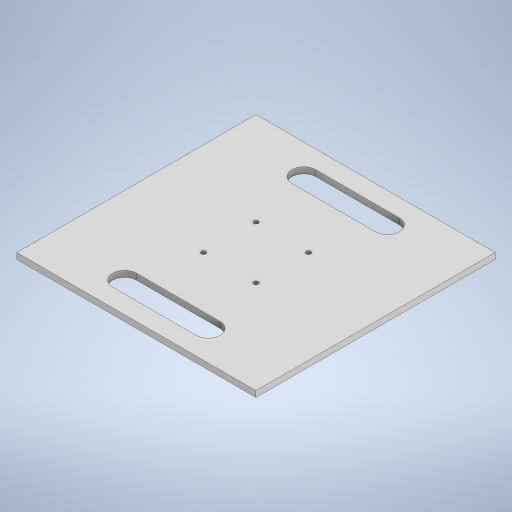
# Autodesk Inventor part: Base myCobot
Saved by Autodesk Inventor 2023.1 (Build 271208000, 208)
## iProperties
Created: 2023-04-03
Part Number: Base myCobot
Material: Generic
Document SubType Name: Modeling
Designer: NITRO 5
Density: 1 g/cm^3
Appearance: Default
Author: NITRO 5
## iProperties of the stored document Base myCobot_3DPrint.ipt
Created: 2023-04-04
Part Number: Base myCobot_3DPrint
Material: Generic
Document SubType Name: Modeling
Designer: NITRO 5
Density: 1 g/cm^3
Appearance: Default
Author: NITRO 5
Autodesk Inventor part; units mm, degrees
ref_plane "YZ Plane" through (0, 0, 0) normal (1, 0, 0) x (0, 1, 0)
ref_plane "XZ Plane" through (0, 0, 0) normal (0, 1, 0) x (-1, 0, 0)
ref_plane "XY Plane" through (0, 0, 0) normal (0, 0, 1) x (1, 0, 0)
sketch "Sketch1" plane through (0, 0, 0) normal (0, 1, 0) x (-1, 0, 0)
  line L0 (-100, 100) -> (100, 100)
  line L1 (100, 100) -> (100, -100)
  line L2 (100, -100) -> (-100, -100)
  line L3 (-100, -100) -> (-100, 100)
  line L4 (-100, 100) -> (100, -100) construction
  line L5 (100, 100) -> (-100, -100) construction
  point P0 (0, 0)
  dimension "d0" = 200
  dimension "d1" = 200
  constraints: 12 end point, 2 midpoint, 2 parallel, 1 horizontal, 1 perpendicular
  measures "d0" distance of L1.end L2.end
  measures "d1" distance of L0.end L1.end
extrude "Extrusion1" add sketch "Sketch1" along normal blind 5
sketch "Sketch6" plane through (0, 0, 0) normal (0, -1, 0) x (1, 0, 0)
  line L0 (-22, 22) -> (22, 22)
  line L1 (22, 22) -> (22, -22)
  line L2 (22, -22) -> (-22, -22)
  line L3 (-22, -22) -> (-22, 22)
  line L4 (-22, 22) -> (22, -22) construction
  line L5 (22, 22) -> (-22, -22) construction
  point P0 (0, 0)
  dimension "d10" = 44
  dimension "d11" = 44
  constraints: 12 end point, 4 coincident, 2 midpoint, 2 parallel, 1 horizontal, 1 perpendicular
  measures "d10" distance of L1.end L2.end
  measures "d11" distance of L0.end L1.end
hole "Hole1" at (22, 0, 22) at (22, 0, -22) at (-22, 0, -22) at (-22, 0, 22) direction (0, 1, 0) diameter 4 depth 49.3
sketch "Sketch7" plane through (0, 0, 0) normal (0, -1, 0) x (1, 0, 0)
  circle A0 centre (-22, 22) radius 2 projected
  circle A1 centre (-22, 22) radius 3
  circle A2 centre (22, 22) radius 2 projected
  circle A3 centre (22, 22) radius 3
  circle A4 centre (-22, -22) radius 2 projected
  circle A5 centre (-22, -22) radius 3
  circle A6 centre (22, -22) radius 3
  point P0 (0, 0)
  dimension "d19" = 6
  dimension "d20" = 6
  dimension "d21" = 6
  dimension "d22" = 6
  constraints: 4 centre point, 3 coincident
  measures "d19" diameter of A1
  measures "d20" diameter of A3
  measures "d21" diameter of A5
  measures "d22" diameter of A6
extrude "Extrusion3" cut sketch "Sketch7" against normal blind 2 contours A0 | A1 | A3 | A5 | A6
sketch "Sketch13" plane through (0, 5, 0) normal (0, 1, 0) x (1, 0, 0)
  line L0 (-35, 75) -> (35, 75) construction
  line L1 (-35, 65) -> (35, 65)
  line L2 (35, 85) -> (-35, 85)
  arc A0 (-35, 85) -> (-35, 65) centre (-35, 75) ccw
  arc A1 (35, 65) -> (35, 85) centre (35, 75) ccw
  line L3 (-35, 75) -> (-35, -100)
  line L4 (-100, -100) -> (100, -100) projected
  line L5 (35, 75) -> (35, -100)
  line L6 (-35, -75) -> (35, -75) construction
  line L7 (-35, -85) -> (35, -85)
  line L8 (35, -65) -> (-35, -65)
  arc A2 (-35, -65) -> (-35, -85) centre (-35, -75) ccw
  arc A3 (35, -85) -> (35, -65) centre (35, -75) ccw
  line L9 (-50, 50) -> (50, 50)
  line L10 (50, 50) -> (50, -50)
  line L11 (50, -50) -> (-50, -50)
  line L12 (-50, -50) -> (-50, 50)
  line L13 (-50, 50) -> (50, -50) construction
  line L14 (50, 50) -> (-50, -50) construction
  line L15 (16.6148, -50) -> (16.6148, -65)
  line L16 (16.6148, -85) -> (16.6148, -100)
  line L17 (31.6927, 50) -> (31.6927, 65)
  point P0 (0, 0)
  point P1 (-100, 100)
  point P2 (0, 75)
  point P3 (0, -75)
  dimension "d56" = 20
  dimension "d59" = 20
  dimension "d60" = 100
  dimension "d61" = 100
  dimension "d62" = 15
  dimension "d64" = 15
  constraints: 38 end point, 12 point on line, 8 point on circle, 8 tangent, 5 parallel, 4 centre point, 4 midpoint, 3 horizontal, 3 perpendicular, 1 vertical
  measures "d56" diameter of A1
  measures "d59" diameter of A3
  measures "d60" distance of L10.end L11.end
  measures "d61" distance of L9.end L10.end
  measures "d62" distance of L15.start L15.end
  measures "d64" distance of L17.start L17.end
extrude "Extrusion5" cut sketch "Sketch13" against normal blind 5 contours A0 L2 A1 L1 | L8 L5 L7 L3 | L3 A2 | A3 L5
sketch "Sketch14" plane through (0, 5, 0) normal (0, 1, 0) x (1, 0, 0)
  point P0 (0, 0)
body "Solid1"
